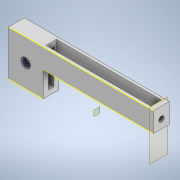
# Autodesk Inventor part: PiezaMovil
Saved by Autodesk Inventor 2020 (Build 240168000, 168)
## iProperties
Created: 2019-09-28
Part Number: PiezaMovil
Material: Genérico
Document SubType Name: Modeling
Designer: Java9
Density: 1 g/cm^3
Appearance: Valor por defecto
Author: Java9
Autodesk Inventor part; units mm, degrees
ref_plane "YZ Plane" through (0, 0, 0) normal (1, 0, 0) x (0, 1, 0)
ref_plane "XZ Plane" through (0, 0, 0) normal (0, 1, 0) x (-1, 0, 0)
ref_plane "XY Plane" through (0, 0, 0) normal (0, 0, 1) x (1, 0, 0)
sketch "Boceto1" plane through (0, 0, 0) normal (0, 0, 1) x (1, 0, 0)
  line L0 (0, 0) -> (130, 0)
  line L1 (130, 0) -> (130, 95)
  line L2 (130, 95) -> (545, 95)
  line L3 (545, 95) -> (545, 170)
  line L4 (545, 170) -> (0, 170)
  line L5 (0, 170) -> (0, 0)
  circle A0 centre (65, 85) radius 10
  dimension "d1" = 95
  dimension "d3" = 75
  dimension "d19" = 20
  constraints: 12 end point, 5 perpendicular, 1 centre point, 1 horizontal
  measures "d1" distance of L0.end L1.end
  measures "d3" distance of L2.end L3.end
  measures "d19" diameter of A0
extrude "Extrusión1" add sketch "Boceto1" along normal blind 60 contours L5 L4 L3 L2 L1 L0 | A0
ref_plane "Plano de trabajo1" through (65, 0, 0) normal (1, 0, 0) x (0, 0, -1)
sketch "Boceto2" plane through (65, 0, 0) normal (1, 0, 0) x (0, 0, -1)
  line L0 (-20, 75) -> (-40, 75)
  line L1 (-40, 75) -> (-40, 20)
  line L2 (0, 0) -> (-60, 0) projected
  line L3 (-40, 20) -> (-20, 20)
  line L4 (-20, 75) -> (-20, 20)
  dimension "d8" = 20
  dimension "d9" = 55
  dimension "d10" = 20
  constraints: 8 end point, 1 perpendicular, 1 vertical
  measures "d8" distance of L0.start L0.end
  measures "d9" distance of L0.end L1.end
  measures "d10" distance of L1.end L3.end
extrude "Extrusión2" cut sketch "Boceto2" along normal blind 400 and the other way blind 200
sketch "Boceto3" plane through (130, 0, 0) normal (1, 0, 0) x (0, 0, -1)
  line L0 (-20, 75) -> (-40, 75) projected
  line L1 (-40, 75) -> (-40, 150)
  line L2 (0, 170) -> (-60, 170) projected
  line L3 (-40, 150) -> (-20, 150)
  line L4 (-20, 150) -> (-20, 75)
  point P0 (0, 0)
  dimension "d15" = 75
  dimension "d16" = 20
  constraints: 6 end point, 3 perpendicular
  measures "d15" distance of L0.end L1.end
  measures "d16" distance of L1.end L3.end
extrude "Extrusión3" cut sketch "Boceto3" along normal mid plane 7000
sketch "Boceto4" plane through (65, 0, 0) normal (1, 0, 0) x (0, 0, -1)
  point P0 (0, 0)
sketch "Boceto5" plane through (0, 0, 60) normal (0, 0, 1) x (1, 0, 0)
  line L0 (130, 95) -> (545, 95) projected
  line L1 (545, 170) -> (0, 170) projected
  line L2 (0, 0) -> (130, 0) projected
  point P0 (65, 85)
hole "Agujero1" at (65, 85, 60) direction (0, 0, -1) diameter 0.2159 end through all thread size "30-318 UNM" class "2B" standard "ANSI Unified Screw Threads"
sketch "Boceto6" plane through (0, 0, 0) normal (-1, 0, 0) x (0, 0, 1)
  line L0 (0, 170) -> (0, 0) projected
  line L1 (40, 95) -> (60, 95) projected
  line L2 (0, 95) -> (60, 95)
  line L3 (0, 95) -> (0, 170)
  line L4 (0, 170) -> (60, 170) projected
  line L5 (60, 170) -> (60, 95)
  constraints: 6 end point, 1 perpendicular, 1 point on line, 1 vertical
extrude "Extrusión4" add sketch "Boceto6" against normal blind 20
ref_plane "Plano de trabajo8" through (272.5, 0, 0) normal (-1, 0, 0) x (0, 0, 1)
sketch "Boceto7" plane through (272.5, 0, 0) normal (-1, 0, 0) x (0, 0, 1)
  line L0 (40, 95) -> (60, 95) projected
  line L1 (0, 75) -> (0, 95) projected
  line L2 (60, 95) -> (0, 95)
  line L3 (0, 95) -> (0, 170)
  line L4 (0, 170) -> (60, 170)
  line L5 (60, 0) -> (60, 95) projected
  line L6 (60, 170) -> (60, 95)
  point P0 (0, 0)
  constraints: 8 end point, 2 perpendicular, 1 collinear, 1 horizontal
extrude "Extrusión5" add sketch "Boceto7" against normal blind 273
sketch "Boceto8" plane through (130, 95, 0) normal (0, -1, 0) x (1, 0, 0)
  line L0 (-130, 60) -> (415.5, 60) projected
  line L1 (415.5, 0) -> (415.5, 60) projected
  line L2 (395.5, 40) -> (395.5, 20)
  line L3 (0, 0) -> (415.5, 0) projected
  line L4 (395.5, 40) -> (142.5, 40)
  line L5 (142.5, 20) -> (0, 20) projected
  line L6 (142.5, 40) -> (142.5, 20)
  line L7 (142.5, 20) -> (395.5, 20)
  point P0 (-130, 0)
  point P1 (415, 60)
  point P2 (415, 0)
  point P3 (415, 20)
  dimension "d35" = 20
  constraints: 8 end point, 3 perpendicular, 1 horizontal
  measures "d35" distance of L2.start L2.end
extrude "Extrusión6" cut sketch "Boceto8" against normal blind 75
sketch "Boceto9" plane through (130, 95, 0) normal (0, -1, 0) x (1, 0, 0)
  line L0 (142.5, 20) -> (142.5, 40) projected
  line L1 (142.5, 20) -> (142.5, 40)
  line L2 (142.5, 40) -> (1, 40)
  line L3 (1, 40) -> (1, 20)
  line L4 (142.5, 20) -> (-110, 20) projected
  line L5 (1, 20) -> (142.5, 20)
  point P0 (-130, 0)
  constraints: 8 end point, 3 perpendicular, 1 vertical
extrude "Extrusión7" cut sketch "Boceto9" against normal blind 75
sketch "Boceto10" plane through (0, 0, 60) normal (0, 0, 1) x (1, 0, 0)
  point P0 (0, 0)
ref_plane "Plano de trabajo9" through (535.5, 0, 0) normal (1, 0, 0) x (0, 0, -1)
sketch "Boceto11" plane through (545.5, 0, 0) normal (1, 0, 0) x (0, 0, -1)
  line L0 (0, 95) -> (-20, 95) projected
  line L1 (0, 170) -> (-60, 170) projected
  line L2 (0, 95) -> (-60, 170)
  line L3 (-60, 84.892) -> (-60, 85.108) projected
  line L4 (0, 170) -> (-60, 85.108)
  circle A0 centre (-30, 127.554) radius 10
  point P0 (0, 0)
  dimension "d40" = 20
  constraints: 4 end point, 1 centre point, 1 midpoint
  measures "d40" diameter of A0
hole "Agujero2" at (545.5, 127.554, 30) direction (-1, 0, 0) diameter 20 end through all
sketch "Boceto12" plane through (0, 0, 60) normal (0, 0, 1) x (1, 0, 0)
  line L0 (0, 170) -> (0, 0) projected
  line L1 (130, 0) -> (130, 95) projected
  line L2 (0, 170) -> (130, 0)
  line L3 (130, 95) -> (130, 170)
  line L4 (130, 170) -> (0, 0)
  circle A0 centre (65, 85) radius 10
  dimension "d48" = 20
  constraints: 6 end point, 1 centre point, 1 midpoint, 1 vertical
  measures "d48" diameter of A0
hole "Agujero3" at (65, 85, 60) direction (0, 0, -1) diameter 20 end through all
extrude "Extrusión8" [suppressed]
hole "Agujero4" at (65, 85, 60) direction (0, 0, -1) diameter 17.8943 end through all thread size "13/16-10 UNC" class "2B" standard "ANSI Unified Screw Threads"
sketch "Boceto13" plane through (0, 170, 60) normal (0, 1, 0) x (1, 0, 0)
  line L0 (131, 40) -> (131, 50)
  line L1 (525.5, 20) -> (525.5, 40) projected
  line L2 (525.5, 40) -> (525.5, 50)
  line L3 (525.5, 50) -> (131, 50)
  line L4 (131, 40) -> (525.5, 40) projected
  line L5 (131, 40) -> (525.5, 40)
  line L6 (525.5, 20) -> (131, 20) projected
  line L7 (131, 20) -> (131, 10)
  line L8 (525.5, 20) -> (525.5, 10)
  line L9 (525.5, 10) -> (131, 10)
  point P0 (0, 60)
  dimension "d65" = 10
  dimension "d66" = 10
  dimension "d67" = 10
  dimension "d68" = 10
  constraints: 14 end point, 4 vertical, 1 horizontal, 1 perpendicular
  measures "d65" distance of L0.start L0.end
  measures "d66" distance of L1.end L2.end
  measures "d67" distance of L6.end L7.end
  measures "d68" distance of L1.start L8.end
extrude "Extrusión9" cut sketch "Boceto13" against normal through all
sketch "Boceto14" plane through (130, 20, 40) normal (0, 0, -1) x (-1, 0, 0)
  circle A0 centre (65, 65) radius 10 projected
  circle A1 centre (65, 65) radius 10
  point P0 (130, -20)
  constraints: 1 centre point, 1 coincident
extrude "Extrusión10" add sketch "Boceto14" along normal blind 40
sketch "Boceto15" plane through (0, 0, 60) normal (0, 0, 1) x (1, 0, 0)
  circle A0 centre (65, 85) radius 10
  circle A1 centre (65, 85) radius 18.123
  point P0 (0, 0)
  dimension "d80" = 36.246
  constraints: 2 centre point, 1 coincident
  measures "d80" diameter of A1
hole "Agujero5" at (65, 85, 60) direction (0, 0, -1) diameter 36.2458 end through all start extended yes thread size "1 9/16-8 UN" class "2B" standard "ANSI Unified Screw Threads"
extrude "Extrusión11" add sketch "Boceto15" along normal mid plane 150 contours A0 | A1
sketch "Boceto16" plane through (0, 0, 0) normal (0, -1, 0) x (1, 0, 0)
  line L0 (0, 60) -> (0, 142)
  line L1 (130, 40) -> (130, 60) projected
  line L2 (130, 60) -> (130, 150)
  line L3 (130, 150) -> (0, 142)
  line L4 (0, 60) -> (130, 60)
  line L5 (131, 50) -> (525.5, 50) projected
  point P0 (0, 0)
  constraints: 8 end point, 2 vertical, 1 parallel
extrude "Extrusión12" cut sketch "Boceto16" against normal blind 150
sketch "Boceto17" plane through (0, 170, 60) normal (0, 1, 0) x (1, 0, 0)
  line L0 (0, 60) -> (130, 60) projected
  line L1 (0, 60) -> (0, 117)
  line L2 (130, 60) -> (130, 106)
  line L3 (0, 60) -> (130, 60)
  line L4 (0, 117) -> (130, 106)
  constraints: 8 end point, 2 vertical, 1 collinear
extrude "Extrusión13" cut sketch "Boceto17" against normal blind 150
sketch "Boceto18" plane through (0, 0, 60) normal (0, 0, 1) x (1, 0, 0)
  circle A0 centre (65, 85) radius 10
  point P0 (0, 0)
  dimension "d87" = 20
  constraints: 1 centre point
  measures "d87" diameter of A0
hole "Agujero6" at (65, 85, 60) direction (0, 0, -1) diameter 36.2458 end through all start extended yes thread size "1 9/16-8 UN" class "2B" standard "ANSI Unified Screw Threads"
